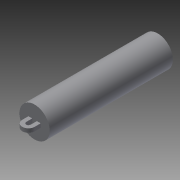
# Autodesk Inventor part: Spring End
Saved by Autodesk Inventor 2014 (Build 180170000, 170)
## iProperties
Created: 2014-01-07
Part Number: Spring End
Material: Generic
Document SubType Name: Modeling
Designer: Andrew Toennies
Density: 1 g/cm^3
Appearance: Default
Author: Andrew Toennies
Autodesk Inventor part; units mm, degrees
ref_plane "YZ Plane" through (0, 0, 0) normal (1, 0, 0) x (0, 1, 0)
ref_plane "XZ Plane" through (0, 0, 0) normal (0, 1, 0) x (-1, 0, 0)
ref_plane "XY Plane" through (0, 0, 0) normal (0, 0, 1) x (1, 0, 0)
sketch "Sketch1" plane through (0, 0, 0) normal (0, 0, 1) x (1, 0, 0)
  circle A0 centre (0, 0) radius 31.2674
  dimension "d0" = 62.5348
  constraints: 1 centre point, 1 coincident
  measures "d0" diameter of A0
extrude "Extrusion1" add sketch "Sketch1" along normal blind 254
sketch "Sketch2" plane through (0, 0, 254) normal (0, 0, 1) x (1, 0, 0)
  circle A0 centre (0, 0) radius 31.2674 projected
  line L0 (-12.7, 3.9624) -> (12.7, 3.9624)
  line L1 (12.7, 3.9624) -> (12.7, -3.9624)
  line L2 (12.7, -3.9624) -> (-12.7, -3.9624)
  line L3 (-12.7, -3.9624) -> (-12.7, 3.9624)
  dimension "d3" = 7.9248
  dimension "d4" = 3.9624
  dimension "d5" = 12.7
  dimension "d6" = 12.7
  constraints: 8 end point, 2 parallel, 1 horizontal, 1 perpendicular
  measures "d3" distance between parallel lines of L2 L0
  measures "d4" distance from line of L2 A0.centre
  measures "d5" distance from line of L3 A0.centre
  measures "d6" distance from line of A0.centre L1
extrude "Extrusion2" add sketch "Sketch2" along normal blind 25.4 contours L0 L1 L2 L3
sketch "Sketch3" plane through (-12.7, 3.9624, 254) normal (0, 1, 0) x (1, 0, 0)
  line L0 (0, 0) -> (25.4, 0) projected
  line L1 (0, 0) -> (0, -25.4) projected
  line L2 (25.4, -25.4) -> (0, -25.4) projected
  line L3 (25.4, 0) -> (25.4, -25.4) projected
  arc A0 (0, -12.7) -> (25.4, -12.7) centre (12.7, -12.7) ccw
  line L4 (7.9248, 0) -> (7.9248, -12.7)
  line L5 (17.4752, 0) -> (17.4752, -12.7)
  arc A1 (7.9248, -12.7) -> (17.4752, -12.7) centre (12.7, -12.7) ccw
  point P0 (12.7, 254)
  dimension "d9" = 7.9248
  constraints: 5 tangent, 4 end point, 4 point on circle, 2 centre point, 2 midpoint, 2 parallel, 2 point on line, 1 coincident
  measures "d9" radial gap between concentric circles of A0 A1
extrude "Extrusion3" cut sketch "Sketch3" against normal blind 25.4 contours L0 L5 A1 L4 | A0 L2 L1 | A0 L3 L2
body "Solid1"
